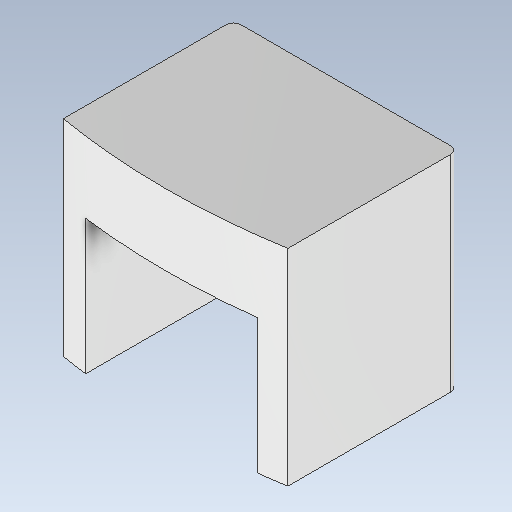
# Autodesk Inventor part: 555_CapAccessory
Saved by Autodesk Inventor 2021 (Build 250183000, 183)
## iProperties
Created: 2021-08-07
Part Number: 555_CapAccessory
Material: アセタール樹脂、白
Document SubType Name: Modeling
Designer: Hagihara Yuya
Density: 1.425 g/cm^3
Appearance: 滑らか - 白
Author: Hagihara Yuya
Autodesk Inventor part; units mm, degrees
ref_plane "YZ Plane" through (0, 0, 0) normal (1, 0, 0) x (0, 1, 0)
ref_plane "XZ Plane" through (0, 0, 0) normal (0, 1, 0) x (-1, 0, 0)
ref_plane "XY Plane" through (0, 0, 0) normal (0, 0, 1) x (1, 0, 0)
sketch "スケッチ1" plane through (0, 0, 0) normal (0, 0, 1) x (1, 0, 0)
  line L0 (3, 13.1) -> (-3, 13.1)
  line L1 (-3, 13.1) -> (-3, 17.9)
  line L2 (-3, 17.9) -> (3, 17.9)
  line L3 (3, 17.9) -> (3, 13.1)
  arc A0 (3, 17.6468) -> (-3, 17.6468) centre (0, 0) ccw
  point P0 (0, 13.1)
  dimension "d0" = 17.9
  dimension "d1" = 6
  dimension "d2" = 4.8
  constraints: 8 end point, 2 parallel, 2 point on circle, 2 point on line, 1 centre point, 1 coincident, 1 horizontal, 1 midpoint, 1 perpendicular, 1 tangent, 1 vertical alignment
  measures "d0" radius of A0
  measures "d1" distance of L0.start L0.end
  measures "d2" distance of L2.end L0.start
extrude "押し出し1" add sketch "スケッチ1" along normal blind 5.5 contours L0 L1 A0 L3
sketch "スケッチ2" plane through (0, 0, 0) normal (0, 0, -1) x (-1, 0, 0)
  line L0 (-2.3, 13.8) -> (2.3, 13.8)
  line L1 (2.3, 13.8) -> (2.3, 17.9)
  line L2 (2.3, 17.9) -> (-2.3, 17.9)
  line L3 (-2.3, 17.9) -> (-2.3, 13.8)
  line L4 (3, 13.1) -> (-3, 13.1) projected
  line L5 (3, 17.6468) -> (3, 13.1) projected
  arc A0 (3, 17.6468) -> (-3, 17.6468) centre (0, 0) ccw projected
  point P0 (0, 13.8)
  point P1 (0, 13.1)
  point P2 (2.3, 17.7516)
  point P3 (-2.3, 17.7516)
  dimension "d5" = 0.7
  dimension "d6" = 0.7
  constraints: 8 end point, 2 midpoint, 2 parallel, 1 horizontal, 1 perpendicular, 1 tangent, 1 vertical alignment
  measures "d5" distance between parallel lines of L4 L0
  measures "d6" distance between parallel lines of L5 L1
extrude "押し出し2" cut sketch "スケッチ2" against normal blind 3.6 contours L3 A0 L1 L0
fillet "フィレット1" radius 0.2 4 edges at (3, 13.1, 2.75) (2.3, 13.8, 1.8) (-2.3, 13.8, 1.8) (-3, 13.1, 2.75)
